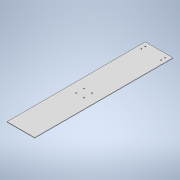
# Autodesk Inventor part: Undercarriage Panel
Saved by Autodesk Inventor 2020 (Build 240168000, 168)
## iProperties
Created: 2021-01-30
Part Number: Undercarriage Panel
Material: Generic
Document SubType Name: Modeling
Designer: magda
Density: 1 g/cm^3
Appearance: Default
Author: magda
Autodesk Inventor part; units mm, degrees
ref_plane "YZ Plane" through (0, 0, 0) normal (1, 0, 0) x (0, 1, 0)
ref_plane "XZ Plane" through (0, 0, 0) normal (0, 1, 0) x (-1, 0, 0)
ref_plane "XY Plane" through (0, 0, 0) normal (0, 0, 1) x (1, 0, 0)
sketch "Sketch1" plane through (0, 0, 0) normal (0, 0, 1) x (1, 0, 0)
  point P0 (0, 0)
sketch "Sketch2" plane through (0, 0, 0) normal (0, 0, 1) x (1, 0, 0)
  line L0 (0, 0) -> (177.8, 0)
  line L1 (177.8, 0) -> (177.8, 3.175)
  line L2 (177.8, 3.175) -> (0, 3.175)
  line L3 (0, 3.175) -> (0, 0)
  dimension "d0" = 177.8
  dimension "d1" = 3.175
  constraints: 8 end point, 2 parallel, 1 horizontal, 1 perpendicular
  measures "d0" distance of L2.end L1.end
  measures "d1" distance between parallel lines of L2 L0
extrude "Extrusion1" add sketch "Sketch2" along normal blind 889
sketch "Sketch3" plane through (0, 3.175, 0) normal (0, 1, 0) x (1, 0, 0)
  line L0 (177.8, 0) -> (0, 0) projected
  line L1 (177.8, 0) -> (177.8, -889) projected
  line L2 (0, 0) -> (0, -889) projected
  point P0 (63.5, -457.2)
  point P1 (114.3, -457.2)
  point P2 (63.5, -508)
  point P3 (114.3, -508)
  dimension "d4" = 457.2
  dimension "d5" = 457.2
  dimension "d6" = 508
  dimension "d7" = 508
  dimension "d8" = 63.5
  dimension "d9" = 63.5
  dimension "d10" = 63.5
  dimension "d11" = 63.5
  measures "d4" distance from line of L0 point (63.5, -457.2)
  measures "d5" distance from line of L0 point (114.3, -457.2)
  measures "d6" distance from line of L0 point (63.5, -508)
  measures "d7" distance from line of point (114.3, -508) L0
  measures "d8" distance from line of point (114.3, -457.2) L1
  measures "d9" distance from line of L1 point (114.3, -508)
  measures "d10" distance from line of L2 point (63.5, -457.2)
  measures "d11" distance from line of L2 point (63.5, -508)
hole "Hole1" at (63.5, 3.175, 457.2) at (63.5, 3.175, 508) at (114.3, 3.175, 508) at (114.3, 3.175, 457.2) direction (0, -1, 0) diameter 6.35 end through all
sketch "Sketch4" plane through (0, 3.175, 0) normal (0, 1, 0) x (1, 0, 0)
  line L0 (177.8, 0) -> (0, 0) projected
  line L1 (0, 0) -> (0, -889) projected
  line L2 (177.8, 0) -> (177.8, -889) projected
  point P0 (25.4, -25.4)
  point P1 (25.4, -50.8)
  point P2 (152.4, -25.4)
  point P3 (152.4, -50.8)
  dimension "d19" = 25.4
  dimension "d20" = 25.4
  dimension "d21" = 25.4
  dimension "d22" = 25.4
  dimension "d23" = 25.4
  dimension "d24" = 25.4
  dimension "d25" = 50.8
  dimension "d26" = 50.8
  measures "d19" distance from line of L0 point (25.4, -25.4)
  measures "d20" distance from line of point (25.4, -25.4) L1
  measures "d21" distance from line of L1 point (25.4, -50.8)
  measures "d22" distance from line of L2 point (152.4, -25.4)
  measures "d23" distance from line of L2 point (152.4, -50.8)
  measures "d24" distance from line of L0 point (152.4, -25.4)
  measures "d25" distance from line of L0 point (152.4, -50.8)
  measures "d26" distance from line of L0 point (25.4, -50.8)
hole "Hole2" at (25.4, 3.175, 25.4) at (25.4, 3.175, 50.8) at (152.4, 3.175, 50.8) at (152.4, 3.175, 25.4) direction (0, -1, 0) diameter 6.35 end through all
body "Solid1"
